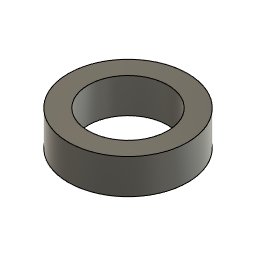
Finger (Autodesk Fusion 360 archive; units mm, degrees)
design "MR128ZZ Ball Bearing"
Autodesk Fusion 360 part; units mm, degrees
sketch "Sketch1" plane through (0, 0, 0) normal (0, 1, 0) x (1, 0, 0)
  circle A0 centre (0, 0) radius 4
  circle A1 centre (0, 0) radius 6
  dimension "d1" = 8
  dimension "d2" = 12
  constraint coincident A0.centre A1.centre
  measures "d1" diameter of A0
  measures "d2" diameter of A1
extrude "Extrude1" add sketch "Sketch1" along normal blind 3.5

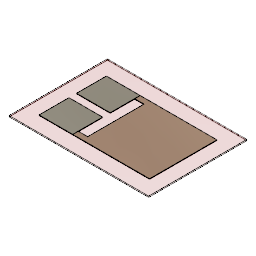
design "BF350 Strain Gauge"
Autodesk Fusion 360 part; units mm, degrees
sketch "Sketch1" plane through (0, 0, 0) normal (0, 0, 1) x (1, 0, 0)
  line L0 (3.725, 2.625) -> (-3.725, 2.625)
  line L1 (-3.725, 2.625) -> (-3.725, -2.625)
  line L2 (-3.725, -2.625) -> (3.725, -2.625)
  line L3 (3.725, -2.625) -> (3.725, 2.625)
  line L4 (3.725, 2.625) -> (-3.725, -2.625) construction
  line L5 (-3.725, 2.625) -> (3.725, -2.625) construction
  line L6 (-0.65, 1.8) -> (2.95, 1.8)
  line L7 (2.95, 1.8) -> (2.95, -1.8)
  line L8 (2.95, -1.8) -> (-0.65, -1.8)
  line L9 (-0.65, -1.8) -> (-0.65, 1.8)
  line L10 (-3.725, 0) -> (3.725, 0) construction
  line L11 (-1.15, 1.8) -> (-2.95, 1.8)
  line L12 (-2.95, 1.8) -> (-2.95, 0.2)
  line L13 (-2.95, 0.2) -> (-1.15, 0.2)
  line L14 (-1.15, 0.2) -> (-1.15, 1.8)
  line L15 (-1.15, 1.5) -> (-0.65, 1.5)
  line L16 (-1.15, 1.8) -> (-0.65, 1.8)
  line L17 (-2.95, 1.8) -> (-3.725, 1.8) construction
  line L18 (2.95, 1.8) -> (3.725, 1.8) construction
  line L19 (-1.15, -1.8) -> (-2.95, -1.8)
  line L20 (-1.15, -0.2) -> (-1.15, -1.8)
  line L21 (-2.95, -0.2) -> (-1.15, -0.2)
  line L22 (-2.95, -1.8) -> (-2.95, -0.2)
  line L23 (-1.15, -1.5) -> (-0.65, -1.5)
  line L24 (-1.15, -1.8) -> (-0.65, -1.8)
  dimension "d1" = 5.25
  dimension "d2" = 7.45
  dimension "d5" = 3.6
  dimension "d6" = 3.6
  dimension "d8" = 1.8
  dimension "d9" = 1.6
  dimension "d11" = 0.3
  dimension "d12" = 0.5
  constraint perpendicular L0 L1
  constraint parallel L0 L2
  constraint horizontal L0
  constraint coincident L4 origin
  constraint coincident L5 origin
  constraint horizontal L6
  constraint vertical L7
  constraint horizontal L8
  constraint vertical L9
  constraint midpoint L1 L10.start
  constraint midpoint L3 L10.end
  constraint symmetric L6 L8 L10
  constraint horizontal L11
  constraint vertical L12
  constraint horizontal L13
  constraint vertical L14
  constraint collinear L6 L11
  constraint perpendicular L0 L3
  constraint coincident L14 L15.start
  constraint coincident L9 L15.end
  constraint perpendicular L9 L15
  constraint coincident L1 L17.end
  constraint perpendicular L1 L17
  constraint coincident L3 L18.end
  constraint perpendicular L3 L18
  constraint equal L17 L18
  constraint symmetric L6.start L10 L8.end
  constraint symmetric L10 L11.start L19.start
  constraint symmetric L10 L11.end L19.end
  constraint symmetric L10 L12.end L21.start
  constraint symmetric L10 L13.end L20.start
  constraint symmetric L10 L15.start L23.start
  constraint symmetric L10 L15.end L23.end
  measures "d1" distance of L0.end L1.end
  measures "d2" distance of L1.end L2.end
  measures "d5" distance of L6.start L6.end
  measures "d6" distance of L6.start L8.end
  measures "d8" distance of L12.end L13.end
  measures "d9" distance of L11.end L12.end
  measures "d11" distance of L15 L16
  measures "d12" distance of L9 L14
extrude "Extrude1" add sketch "Sketch1" against normal blind 0.07 contours L0 L1 L2 L3 | L6 L7 L8 L9 | L9 L14 L15 L16 | L11 L12 L13 L14 | L9 L20 L23 L24 | L19 L20 L21 L22 makes body 1
extrude "Extrude2" add sketch "Sketch1" against normal blind 0.03 separate body contours L6 L7 L8 L9 | L9 L14 L15 L16 | L9 L20 L23 L24 makes body 2
extrude "Extrude3" add sketch "Sketch1" against normal blind 0.03 separate body contours L11 L12 L13 L14 | L19 L20 L21 L22 makes body 3 at (-1.75, -1.2667, 0) makes body 4 at (-2.35, 1.2667, 0)
combine "Combine1" operation cut target body 1 tool bodies 2 4 3 keep tools
